Autodesk Inventor part; units mm, degrees
(part 6 of 8)
  spline S105 degree 3 poles (-3.7054, -6.6544) (-3.6945, -6.6546) (-3.6729, -6.6551) (-3.6415, -6.6595) (-3.6115, -6.6662) (-3.5832, -6.6758) (-3.5566, -6.6886) (-3.5316, -6.7039) (-3.5079, -6.7217) (-3.4866, -6.7426) (-3.467, -6.765) (-3.4501, -6.7888) (-3.4357, -6.8135) (-3.4236, -6.8391) (-3.4148, -6.8659) (-3.408, -6.8935) (-3.4042, -6.9223) (-3.4036, -6.9417) (-3.4033, -6.9516) knots 0 0 0 0 0.069475 0.136517 0.200789 0.26383 0.325735 0.387291 0.449509 0.512968 0.576275 0.63758 0.697903 0.757172 0.816599 0.876653 0.93729 1 1 1 1
  spline S106 degree 3 poles (-3.4033, -6.9516) (-3.4038, -6.9656) (-3.4048, -6.9932) (-3.413, -7.0337) (-3.4258, -7.0731) (-3.4412, -7.1047) (-3.4568, -7.1302) (-3.4708, -7.1512) (-3.4872, -7.1738) (-3.5063, -7.1979) (-3.5276, -7.2238) (-3.5513, -7.2514) (-3.5776, -7.2803) (-3.5961, -7.3001) (-3.6057, -7.3104) knots 0 0 0 0 0.098702 0.195672 0.292422 0.391343 0.444462 0.504229 0.570352 0.642546 0.722288 0.807921 0.90047 1 1 1 1
  line L71 (-3.6057, -7.3104) -> (-3.8559, -7.5774)
  line L72 (-3.8559, -7.5774) -> (-3.3905, -7.5774)
  line L73 (-3.3905, -7.5774) -> (-3.3905, -7.68)
  line L74 (-3.3905, -7.68) -> (-4.07, -7.68)
  line L75 (-4.07, -7.68) -> (-3.6822, -7.2661)
  spline S107 degree 3 poles (-3.6822, -7.2661) (-3.6727, -7.2563) (-3.6546, -7.2373) (-3.6289, -7.2097) (-3.6059, -7.1841) (-3.5853, -7.1605) (-3.5677, -7.1386) (-3.552, -7.1191) (-3.5394, -7.1012) (-3.5258, -7.0804) (-3.5126, -7.055) (-3.5012, -7.024) (-3.4943, -6.9921) (-3.4935, -6.9705) (-3.4931, -6.9596) knots 0 0 0 0 0.110803 0.212829 0.306101 0.390647 0.466924 0.534481 0.593587 0.644557 0.7362 0.825024 0.911986 1 1 1 1
  line L76 (-3.0444, -10.22) -> (-3.0572, -10.22)
  line L77 (-3.0572, -10.22) -> (-3.4803, -9.22)
  line L78 (-3.4803, -9.22) -> (-3.3841, -9.22)
  line L79 (-3.3841, -9.22) -> (-3.0508, -10.0081)
  line L80 (-3.0508, -10.0081) -> (-2.7174, -9.22)
  line L81 (-2.7174, -9.22) -> (-2.6213, -9.22)
  line L82 (-2.6213, -9.22) -> (-3.0444, -10.22)
  spline S108 degree 3 poles (-6.6469, -12.2726) (-6.6471, -12.285) (-6.6475, -12.3093) (-6.6506, -12.3452) (-6.6553, -12.3801) (-6.6624, -12.4137) (-6.6711, -12.4463) (-6.6822, -12.4777) (-6.695, -12.5081) (-6.7099, -12.5371) (-6.7262, -12.5645) (-6.7437, -12.5904) (-6.7624, -12.6143) (-6.7825, -12.6364) (-6.8036, -12.6566) (-6.826, -12.675) (-6.8496, -12.6913) (-6.8745, -12.7062) (-6.9013, -12.7192) (-6.9304, -12.7302) (-6.9622, -12.7393) (-6.9964, -12.7469) (-7.0331, -12.7529) (-7.0723, -12.7569) (-7.1141, -12.7596) (-7.1428, -12.7599) (-7.1575, -12.76) knots 0 0 0 0 0.046081 0.090807 0.134295 0.177024 0.218823 0.260244 0.30108 0.341614 0.381583 0.42012 0.458075 0.494738 0.531195 0.566934 0.602713 0.638327 0.674853 0.713467 0.754442 0.797815 0.843989 0.893072 0.944963 1 1 1 1
  line L83 (-7.1575, -12.76) -> (-7.4674, -12.76)
  line L84 (-7.4674, -12.76) -> (-7.4674, -11.76)
  line L85 (-7.4674, -11.76) -> (-7.2655, -11.76)
  spline S109 degree 3 poles (-7.2655, -11.76) (-7.248, -11.7601) (-7.214, -11.7604) (-7.165, -11.7619) (-7.1196, -11.7647) (-7.0781, -11.7687) (-7.0402, -11.7736) (-7.0062, -11.7797) (-6.9758, -11.7869) (-6.9571, -11.7931) (-6.9482, -11.7961) knots 0 0 0 0 0.164289 0.317406 0.458844 0.589367 0.707831 0.81577 0.91288 1 1 1 1
  spline S110 degree 3 poles (-6.9482, -11.7961) (-6.9366, -11.8005) (-6.9138, -11.8092) (-6.8812, -11.8256) (-6.8505, -11.8443) (-6.8216, -11.8651) (-6.7951, -11.8888) (-6.7699, -11.9142) (-6.7472, -11.9424) (-6.7264, -11.9727) (-6.7076, -12.0048) (-6.6913, -12.0386) (-6.6777, -12.0739) (-6.6664, -12.1107) (-6.6576, -12.1491) (-6.6515, -12.189) (-6.6475, -12.2303) (-6.6471, -12.2584) (-6.6469, -12.2726) knots 0 0 0 0 0.061545 0.121694 0.181155 0.239875 0.298702 0.357647 0.417605 0.478494 0.540407 0.602345 0.665004 0.728559 0.793651 0.860534 0.929236 1 1 1 1
  line L86 (-8.4033, -11.9747) -> (-8.4033, -12.76)
  line L87 (-8.4033, -12.76) -> (-8.4931, -12.76)
  line L88 (-8.4931, -12.76) -> (-8.4931, -11.76)
  line L89 (-8.4931, -11.76) -> (-8.4742, -11.76)
  line L90 (-8.4742, -11.76) -> (-7.8136, -12.5471)
  line L91 (-7.8136, -12.5471) -> (-7.8136, -11.76)
  line L92 (-7.8136, -11.76) -> (-7.7238, -11.76)
  line L93 (-7.7238, -11.76) -> (-7.7238, -12.76)
  line L94 (-7.7238, -12.76) -> (-7.7443, -12.76)
  line L95 (-7.7443, -12.76) -> (-8.4033, -11.9747)
  spline S111 degree 3 poles (-9.7495, -12.2596) (-9.7493, -12.2478) (-9.749, -12.2245) (-9.7454, -12.1898) (-9.7401, -12.1557) (-9.7324, -12.1222) (-9.7226, -12.0894) (-9.7105, -12.0572) (-9.6963, -12.0256) (-9.6799, -11.9948) (-9.6616, -11.9651) (-9.6417, -11.9369) (-9.62, -11.9104) (-9.5968, -11.8855) (-9.5718, -11.8624) (-9.5453, -11.841) (-9.5172, -11.8211) (-9.4875, -11.8031) (-9.4567, -11.7869) (-9.4246, -11.7728) (-9.3915, -11.7611) (-9.3575, -11.7511) (-9.3224, -11.7438) (-9.2864, -11.7384) (-9.2494, -11.7348) (-9.2243, -11.7345) (-9.2116, -11.7344) knots 0 0 0 0 0.042039 0.083544 0.124643 0.165303 0.206171 0.246971 0.288329 0.329987 0.371797 0.412738 0.453459 0.494001 0.534381 0.574952 0.615892 0.65725 0.699007 0.740486 0.782325 0.824567 0.867041 0.9105 0.954619 1 1 1 1
  spline S112 degree 3 poles (-9.2116, -11.7344) (-9.2013, -11.7345) (-9.1807, -11.7349) (-9.1502, -11.7371) (-9.1201, -11.7407) (-9.0905, -11.7457) (-9.0613, -11.7524) (-9.0327, -11.7604) (-9.0044, -11.7697) (-8.9766, -11.7809) (-8.9491, -11.7935) (-8.9218, -11.8077) (-8.8947, -11.8238) (-8.8679, -11.8417) (-8.841, -11.8613) (-8.8146, -11.8829) (-8.7881, -11.9058) (-8.771, -11.9223) (-8.7623, -11.9307) knots 0 0 0 0 0.061617 0.122179 0.182216 0.241864 0.30096 0.359969 0.419033 0.478069 0.537993 0.59896 0.661321 0.725248 0.79122 0.858746 0.928318 1 1 1 1
  line L96 (-8.7623, -11.9307) -> (-8.8392, -12.0036)
  spline S113 degree 3 poles (-8.8392, -12.0036) (-8.8532, -11.9905) (-8.8807, -11.9646) (-8.9255, -11.931) (-8.9723, -11.9023) (-9.0208, -11.8789) (-9.0698, -11.8602) (-9.1186, -11.8469) (-9.1668, -11.8384) (-9.1988, -11.8374) (-9.2146, -11.8369) knots 0 0 0 0 0.136144 0.269043 0.398517 0.5271 0.652283 0.77168 0.887495 1 1 1 1
  spline S114 degree 3 poles (-9.2146, -11.8369) (-9.2243, -11.837) (-9.2437, -11.8373) (-9.2724, -11.8403) (-9.3009, -11.8446) (-9.329, -11.8509) (-9.3568, -11.8588) (-9.3842, -11.8688) (-9.4112, -11.8804) (-9.4376, -11.8938) (-9.4633, -11.9085) (-9.4875, -11.9248) (-9.5105, -11.9421) (-9.5317, -11.961) (-9.5514, -11.9812) (-9.5699, -12.0024) (-9.5867, -12.0251) (-9.6019, -12.0489) (-9.6154, -12.0734) (-9.6274, -12.0984) (-9.6374, -12.1237) (-9.6453, -12.1495) (-9.6519, -12.1755) (-9.6565, -12.2018) (-9.6591, -12.2286) (-9.6595, -12.2466) (-9.6597, -12.2556) knots 0 0 0 0 0.042841 0.085571 0.127719 0.170068 0.212787 0.255482 0.298877 0.342861 0.386528 0.429532 0.471886 0.513729 0.555082 0.596535 0.63812 0.679822 0.721331 0.761888 0.802199 0.841806 0.88106 0.920633 0.960101 1 1 1 1
  spline S115 degree 3 poles (-9.6597, -12.2556) (-9.6595, -12.2648) (-9.6591, -12.2832) (-9.6563, -12.3107) (-9.6512, -12.3378) (-9.6444, -12.3645) (-9.6358, -12.391) (-9.6251, -12.4171) (-9.6125, -12.4428) (-9.5978, -12.4679) (-9.5818, -12.4923) (-9.5638, -12.5154) (-9.5447, -12.5373) (-9.5238, -12.5576) (-9.5017, -12.5768) (-9.4778, -12.5945) (-9.4526, -12.6109) (-9.4261, -12.6259) (-9.3984, -12.6393) (-9.3701, -12.6512) (-9.3409, -12.661) (-9.3111, -12.6689) (-9.2807, -12.6755) (-9.2496, -12.6797) (-9.2179, -12.6827) (-9.1965, -12.683) (-9.1858, -12.6831) knots 0 0 0 0 0.038994 0.077882 0.116652 0.155416 0.194618 0.234261 0.274547 0.315667 0.35702 0.398083 0.439098 0.479833 0.521274 0.562841 0.605292 0.648409 0.691727 0.735149 0.778369 0.821661 0.865524 0.909731 0.954523 1 1 1 1
  spline S116 degree 3 poles (-9.1858, -12.6831) (-9.1728, -12.6828) (-9.1474, -12.6823) (-9.1099, -12.6781) (-9.074, -12.6717) (-9.0396, -12.6622) (-9.0068, -12.6501) (-8.9754, -12.6355) (-8.9457, -12.6179) (-8.9175, -12.598) (-8.8916, -12.5759) (-8.8682, -12.552) (-8.8477, -12.5265) (-8.8299, -12.4994) (-8.8151, -12.4707) (-8.803, -12.4404) (-8.7937, -12.4085) (-8.7899, -12.3865) (-8.7879, -12.3754) knots 0 0 0 0 0.07063 0.138694 0.204918 0.269441 0.332636 0.395302 0.457764 0.520657 0.582852 0.643315 0.70258 0.760908 0.81949 0.878269 0.938491 1 1 1 1
  line L97 (-8.7879, -12.3754) -> (-9.1213, -12.3754)
  line L98 (-9.1213, -12.3754) -> (-9.1213, -12.2728)
  line L99 (-9.1213, -12.2728) -> (-8.6982, -12.2728)
  spline S117 degree 3 poles (-8.6982, -12.2728) (-8.6987, -12.2919) (-8.6996, -12.3294) (-8.7063, -12.3839) (-8.7171, -12.4354) (-8.7319, -12.484) (-8.751, -12.5295) (-8.7743, -12.572) (-8.802, -12.6113) (-8.8333, -12.6476) (-8.8684, -12.68) (-8.9064, -12.7084) (-8.9473, -12.7324) (-8.9912, -12.7519) (-9.0378, -12.7671) (-9.0872, -12.7779) (-9.1395, -12.7844) (-9.1753, -12.7852) (-9.1936, -12.7856) knots 0 0 0 0 0.071272 0.139493 0.204635 0.267406 0.328446 0.388397 0.447734 0.507392 0.566768 0.625478 0.684067 0.743248 0.804033 0.866499 0.931723 1 1 1 1
  spline S118 degree 3 poles (-9.1936, -12.7856) (-9.2049, -12.7855) (-9.2272, -12.7852) (-9.26, -12.7829) (-9.292, -12.7794) (-9.3231, -12.7741) (-9.3533, -12.7676) (-9.3827, -12.7593) (-9.4111, -12.7497) (-9.4388, -12.7387) (-9.4655, -12.726) (-9.4912, -12.7119) (-9.5161, -12.6965) (-9.5401, -12.6795) (-9.5633, -12.661) (-9.5855, -12.641) (-9.6068, -12.6195) (-9.6202, -12.6042) (-9.6269, -12.5965) knots 0 0 0 0 0.069237 0.136557 0.202094 0.266464 0.329769 0.391879 0.453271 0.514115 0.57439 0.634142 0.693923 0.754152 0.81447 0.875661 0.937348 1 1 1 1
  spline S119 degree 3 poles (-9.6269, -12.5965) (-9.6367, -12.5843) (-9.656, -12.5602) (-9.681, -12.5214) (-9.7022, -12.4813) (-9.7195, -12.4397) (-9.7329, -12.3967) (-9.7426, -12.3522) (-9.7483, -12.3064) (-9.7491, -12.2753) (-9.7495, -12.2596) knots 0 0 0 0 0.127896 0.253668 0.376738 0.499344 0.621999 0.745699 0.871345 1 1 1 1
  line L100 (-2.9033, -12.76) -> (-2.9033, -11.8626)
  line L101 (-2.9033, -11.8626) -> (-3.1213, -11.8626)
  line L102 (-3.1213, -11.8626) -> (-3.1213, -11.76)
  line L103 (-3.1213, -11.76) -> (-2.5956, -11.76)
  line L104 (-2.5956, -11.76) -> (-2.5956, -11.8626)
  line L105 (-2.5956, -11.8626) -> (-2.8136, -11.8626)
  line L106 (-2.8136, -11.8626) -> (-2.8136, -12.76)
  line L107 (-2.8136, -12.76) -> (-2.9033, -12.76)
  spline S120 degree 3 poles (-3.211, -12.515) (-3.2112, -12.524) (-3.2116, -12.5417) (-3.2159, -12.5678) (-3.2221, -12.5931) (-3.2316, -12.6174) (-3.2431, -12.641) (-3.2577, -12.6634) (-3.2746, -12.6851) (-3.2941, -12.7054) (-3.3154, -12.7241) (-3.3378, -12.7407) (-3.3616, -12.7546) (-3.3864, -12.7659) (-3.4124, -12.7747) (-3.4395, -12.7811) (-3.4677, -12.785) (-3.4869, -12.7854) (-3.4967, -12.7856) knots 0 0 0 0 0.061484 0.121775 0.18092 0.240256 0.300114 0.361146 0.423501 0.488669 0.553954 0.617581 0.680238 0.742187 0.804663 0.868259 0.93302 1 1 1 1
  spline S121 degree 3 poles (-3.4967, -12.7856) (-3.5042, -12.7855) (-3.5192, -12.7852) (-3.5414, -12.7826) (-3.5632, -12.779) (-3.5842, -12.7732) (-3.6048, -12.7663) (-3.6249, -12.7576) (-3.6444, -12.7473) (-3.6635, -12.7355) (-3.6821, -12.7218) (-3.7001, -12.7058) (-3.718, -12.688) (-3.7353, -12.6679) (-3.7524, -12.6458) (-3.769, -12.6215) (-3.7853, -12.5952) (-3.7955, -12.5766) (-3.8008, -12.5671) knots 0 0 0 0 0.057208 0.113696 0.169178 0.224159 0.27872 0.333794 0.389241 0.445822 0.503704 0.564294 0.627975 0.695038 0.765373 0.839611 0.917538 1 1 1 1
  line L108 (-3.8008, -12.5671) -> (-3.7162, -12.5164)
  spline S122 degree 3 poles (-3.7162, -12.5164) (-3.7084, -12.5296) (-3.6933, -12.5548) (-3.6682, -12.5889) (-3.6421, -12.6178) (-3.615, -12.6415) (-3.5869, -12.6601) (-3.5577, -12.6733) (-3.5275, -12.6816) (-3.5069, -12.6826) (-3.4967, -12.6831) knots 0 0 0 0 0.159004 0.304646 0.438547 0.562322 0.677433 0.786897 0.893611 1 1 1 1
  spline S123 degree 3 poles (-3.4967, -12.6831) (-3.4879, -12.6828) (-3.4705, -12.6823) (-3.4449, -12.6777) (-3.4201, -12.6706) (-3.3965, -12.6603) (-3.3745, -12.6479) (-3.3551, -12.633) (-3.3384, -12.6162) (-3.3248, -12.5976) (-3.3143, -12.5775) (-3.3063, -12.5568) (-3.3018, -12.5354) (-3.3011, -12.5209) (-3.3008, -12.5136) knots 0 0 0 0 0.091264 0.18093 0.270088 0.360156 0.448343 0.532666 0.613834 0.693982 0.772716 0.849335 0.923967 1 1 1 1
  spline S124 degree 3 poles (-3.3008, -12.5136) (-3.3012, -12.5053) (-3.302, -12.4884) (-3.3093, -12.4634) (-3.3207, -12.4387) (-3.3312, -12.4234) (-3.3366, -12.4154) knots 0 0 0 0 0.234723 0.477158 0.728556 1 1 1 1
  spline S125 degree 3 poles (-3.3366, -12.4154) (-3.3411, -12.4097) (-3.3505, -12.3977) (-3.3667, -12.3798) (-3.3856, -12.3613) (-3.4067, -12.3416) (-3.4308, -12.3215) (-3.457, -12.3001) (-3.486, -12.2782) (-3.5064, -12.2636) (-3.5169, -12.256) knots 0 0 0 0 0.090279 0.18953 0.299198 0.418926 0.548376 0.688136 0.839084 1 1 1 1
  spline S126 degree 3 poles (-3.5169, -12.256) (-3.5274, -12.2485) (-3.5476, -12.2342) (-3.5757, -12.2129) (-3.6008, -12.1935) (-3.6229, -12.1757) (-3.6419, -12.1595) (-3.6579, -12.1451) (-3.6706, -12.1322) (-3.6776, -12.1238) (-3.6808, -12.12) knots 0 0 0 0 0.181535 0.347082 0.495568 0.628357 0.74552 0.845831 0.930782 1 1 1 1
  spline S127 degree 3 poles (-3.6808, -12.12) (-3.6852, -12.1141) (-3.6939, -12.1025) (-3.7054, -12.0844) (-3.7151, -12.0659) (-3.7228, -12.0469) (-3.7292, -12.0277) (-3.7335, -12.008) (-3.7362, -11.988) (-3.7365, -11.9745) (-3.7367, -11.9677) knots 0 0 0 0 0.133507 0.262559 0.388264 0.512667 0.633722 0.755394 0.877553 1 1 1 1
  spline S128 degree 3 poles (-3.7367, -11.9677) (-3.7363, -11.9572) (-3.7356, -11.9362) (-3.7293, -11.9056) (-3.7195, -11.8764) (-3.7057, -11.8489) (-3.6879, -11.8238) (-3.6673, -11.8008) (-3.6428, -11.7814) (-3.6159, -11.7645) (-3.5864, -11.7512) (-3.5556, -11.7412) (-3.5233, -11.7356) (-3.5014, -11.7348) (-3.4903, -11.7344) knots 0 0 0 0 0.083785 0.16578 0.24628 0.327461 0.408797 0.489715 0.571376 0.655523 0.741019 0.826547 0.911989 1 1 1 1
  spline S129 degree 3 poles (-3.4903, -11.7344) (-3.4785, -11.7348) (-3.4551, -11.7356) (-3.4206, -11.7426) (-3.3874, -11.7542) (-3.3607, -11.7674) (-3.3398, -11.7806) (-3.3239, -11.7926) (-3.3077, -11.8064) (-3.2912, -11.8221) (-3.2747, -11.8398) (-3.2578, -11.8593) (-3.2406, -11.8806) (-3.2295, -11.8958) (-3.2238, -11.9036) knots 0 0 0 0 0.107233 0.213252 0.31883 0.426794 0.483646 0.543604 0.608308 0.677127 0.750686 0.828713 0.91219 1 1 1 1
  line L109 (-3.2238, -11.9036) -> (-3.305, -11.9651)
  spline S130 degree 3 poles (-3.305, -11.9651) (-3.3099, -11.9588) (-3.3193, -11.9467) (-3.3336, -11.9296) (-3.3471, -11.9141) (-3.3604, -11.9006) (-3.3728, -11.8884) (-3.3849, -11.8779) (-3.3964, -11.8692) (-3.4108, -11.8598) (-3.4291, -11.8505) (-3.4519, -11.8426) (-3.4758, -11.8379) (-3.4921, -11.8372) (-3.5003, -11.8369) knots 0 0 0 0 0.098469 0.189629 0.274184 0.352183 0.423199 0.488551 0.548473 0.60144 0.701198 0.799592 0.898545 1 1 1 1
  spline S131 degree 3 poles (-3.5003, -11.8369) (-3.5106, -11.8373) (-3.5305, -11.8379) (-3.5588, -11.8452) (-3.5843, -11.8567) (-3.6062, -11.8728) (-3.6244, -11.8919) (-3.6375, -11.9138) (-3.6455, -11.938) (-3.6464, -11.9549) (-3.6469, -11.9635) knots 0 0 0 0 0.143073 0.275903 0.402371 0.528414 0.650356 0.765895 0.880774 1 1 1 1
  spline S132 degree 3 poles (-3.6469, -11.9635) (-3.6468, -11.9689) (-3.6466, -11.9796) (-3.6435, -11.9955) (-3.6394, -12.0113) (-3.633, -12.0269) (-3.6242, -12.0428) (-3.6127, -12.0591) (-3.5981, -12.076) (-3.5869, -12.0869) (-3.581, -12.0927) knots 0 0 0 0 0.107285 0.214746 0.322939 0.434116 0.553412 0.686073 0.834256 1 1 1 1
  spline S133 degree 3 poles (-3.581, -12.0927) (-3.5788, -12.0947) (-3.5736, -12.0993) (-3.5641, -12.1069) (-3.5516, -12.1163) (-3.5363, -12.1279) (-3.518, -12.1413) (-3.4967, -12.1565) (-3.4727, -12.1738) (-3.4556, -12.1859) (-3.4466, -12.1923) knots 0 0 0 0 0.052594 0.124952 0.218094 0.333502 0.468789 0.624938 0.801683 1 1 1 1
  spline S134 degree 3 poles (-3.4466, -12.1923) (-3.4357, -12.2002) (-3.4147, -12.2155) (-3.3848, -12.2385) (-3.3577, -12.2609) (-3.3333, -12.2828) (-3.3113, -12.3038) (-3.2921, -12.3242) (-3.2753, -12.3439) (-3.2572, -12.3693) (-3.2388, -12.4003) (-3.223, -12.4384) (-3.213, -12.4766) (-3.2117, -12.5023) (-3.211, -12.515) knots 0 0 0 0 0.096972 0.187773 0.272396 0.351321 0.424335 0.491909 0.554233 0.611268 0.716348 0.81454 0.908495 1 1 1 1
  spline S135 degree 3 poles (4.429, 5.5196) (4.4288, 5.5043) (4.4284, 5.4745) (4.4265, 5.4309) (4.4228, 5.3898) (4.4182, 5.351) (4.4118, 5.3147) (4.4039, 5.2808) (4.3952, 5.2491) (4.3843, 5.2198) (4.3725, 5.1927) (4.3596, 5.1674) (4.3458, 5.1436) (4.3308, 5.1216) (4.3148, 5.1012) (4.2975, 5.0828) (4.2793, 5.0659) (4.26, 5.0509) (4.2399, 5.0377) (4.2193, 5.0259) (4.198, 5.0164) (4.1763, 5.0083) (4.154, 5.002) (4.131, 4.9977) (4.1076, 4.9947) (4.0918, 4.9945) (4.0838, 4.9944) knots 0 0 0 0 0.065063 0.126773 0.185516 0.240765 0.29298 0.34225 0.388919 0.432776 0.474628 0.514775 0.553606 0.591426 0.628028 0.663804 0.698984 0.733591 0.767628 0.801208 0.834264 0.866981 0.89972 0.932702 0.966176 1 1 1 1
  spline S136 degree 3 poles (4.0838, 4.9944) (4.0759, 4.9945) (4.0604, 4.9948) (4.0373, 4.9975) (4.015, 5.0018) (3.9932, 5.008) (3.9718, 5.0155) (3.9512, 5.0252) (3.9311, 5.0364) (3.9116, 5.0492) (3.8931, 5.0639) (3.8753, 5.0801) (3.8589, 5.0983) (3.8435, 5.1182) (3.829, 5.1395) (3.8156, 5.1626) (3.8032, 5.1874) (3.7919, 5.2141) (3.7818, 5.243) (3.7729, 5.2745) (3.7659, 5.3088) (3.7599, 5.3457) (3.7551, 5.3853) (3.7518, 5.4277) (3.7498, 5.4728) (3.7496, 5.5037) (3.7495, 5.5196) knots 0 0 0 0 0.033787 0.066622 0.099285 0.131361 0.163585 0.196104 0.228902 0.262158 0.295991 0.330218 0.36506 0.400951 0.43762 0.475708 0.515381 0.556414 0.599765 0.646424 0.696431 0.749782 0.806573 0.867436 0.931887 1 1 1 1
  spline S137 degree 3 poles (3.7495, 5.5196) (3.7496, 5.5356) (3.7498, 5.5668) (3.7518, 5.6121) (3.7552, 5.6547) (3.7598, 5.6944) (3.7654, 5.7314) (3.7729, 5.7655) (3.7814, 5.7968) (3.7913, 5.8255) (3.8024, 5.852) (3.8145, 5.8766) (3.8281, 5.8995) (3.8424, 5.921) (3.8579, 5.9407) (3.8743, 5.9589) (3.8921, 5.9751) (3.9108, 5.99) (3.9306, 6.0029) (3.9507, 6.0144) (3.9715, 6.0241) (3.993, 6.0318) (4.0149, 6.0382) (4.0373, 6.0425) (4.0604, 6.0452) (4.0759, 6.0455) (4.0838, 6.0456) knots 0 0 0 0 0.068595 0.133246 0.194313 0.251279 0.304513 0.354235 0.400481 0.443411 0.484015 0.523252 0.561042 0.5979 0.633518 0.668314 0.702496 0.736685 0.770293 0.803437 0.835913 0.86846 0.900847 0.933467 0.966258 1 1 1 1
  spline S138 degree 3 poles (4.0838, 6.0456) (4.0918, 6.0455) (4.1076, 6.0452) (4.131, 6.0426) (4.1538, 6.0381) (4.176, 6.0319) (4.1978, 6.0241) (4.2189, 6.0144) (4.2395, 6.003) (4.2593, 5.9897) (4.2785, 5.9749) (4.2967, 5.9581) (4.3137, 5.9395) (4.3299, 5.9194) (4.3448, 5.8973) (4.359, 5.8737) (4.3716, 5.848) (4.3838, 5.8208) (4.3944, 5.7913) (4.4039, 5.7597) (4.4116, 5.7255) (4.418, 5.689) (4.4229, 5.65) (4.4265, 5.6087) (4.4284, 5.5649) (4.4288, 5.535) (4.429, 5.5196) knots 0 0 0 0 0.033788 0.067194 0.099862 0.132567 0.165151 0.197913 0.231319 0.265083 0.299255 0.334399 0.369943 0.406284 0.444064 0.482998 0.523354 0.565537 0.609613 0.656391 0.705885 0.758325 0.813832 0.872795 0.934722 1 1 1 1
  line L110 (4.9674, 5.02) -> (4.9546, 5.02)
  line L111 (4.9546, 5.02) -> (4.5315, 6.02)
  line L112 (4.5315, 6.02) -> (4.6277, 6.02)
  line L113 (4.6277, 6.02) -> (4.961, 5.2319)
  line L114 (4.961, 5.2319) -> (5.2944, 6.02)
  line L115 (5.2944, 6.02) -> (5.3905, 6.02)
  line L116 (5.3905, 6.02) -> (4.9674, 5.02)
  spline S139 degree 3 poles (5.7495, 2.9674) (5.7493, 2.955) (5.749, 2.9307) (5.7458, 2.8948) (5.7412, 2.8599) (5.734, 2.8263) (5.7253, 2.7937) (5.7142, 2.7623) (5.7014, 2.7319) (5.6866, 2.7029) (5.6702, 2.6755) (5.6527, 2.6496) (5.634, 2.6257) (5.614, 2.6036) (5.5928, 2.5834) (5.5704, 2.565) (5.5468, 2.5487) (5.5219, 2.5338) (5.4951, 2.5208) (5.466, 2.5098) (5.4342, 2.5007) (5.4001, 2.4931) (5.3633, 2.4871) (5.3241, 2.4831) (5.2823, 2.4804) (5.2536, 2.4801) (5.2389, 2.48) knots 0 0 0 0 0.046081 0.090807 0.134295 0.177024 0.218823 0.260244 0.30108 0.341614 0.381583 0.42012 0.458075 0.494738 0.531195 0.566934 0.602713 0.638327 0.674853 0.713467 0.754442 0.797815 0.843989 0.893072 0.944963 1 1 1 1
  line L117 (5.2389, 2.48) -> (4.929, 2.48)
  line L118 (4.929, 2.48) -> (4.929, 3.48)
  line L119 (4.929, 3.48) -> (5.1309, 3.48)
  spline S140 degree 3 poles (5.1309, 3.48) (5.1485, 3.4799) (5.1824, 3.4796) (5.2314, 3.4781) (5.2768, 3.4753) (5.3183, 3.4713) (5.3562, 3.4664) (5.3902, 3.4603) (5.4207, 3.4531) (5.4394, 3.4469) (5.4482, 3.4439) knots 0 0 0 0 0.164289 0.317406 0.458844 0.589367 0.707831 0.81577 0.91288 1 1 1 1
  spline S141 degree 3 poles (5.4482, 3.4439) (5.4598, 3.4395) (5.4827, 3.4308) (5.5152, 3.4144) (5.5459, 3.3957) (5.5748, 3.3749) (5.6013, 3.3512) (5.6265, 3.3258) (5.6492, 3.2976) (5.67, 3.2673) (5.6888, 3.2352) (5.7052, 3.2014) (5.7187, 3.1661) (5.73, 3.1293) (5.7388, 3.0909) (5.7449, 3.051) (5.7489, 3.0097) (5.7493, 2.9816) (5.7495, 2.9674) knots 0 0 0 0 0.061545 0.121694 0.181155 0.239875 0.298702 0.357647 0.417605 0.478494 0.540407 0.602345 0.665004 0.728559 0.793651 0.860534 0.929236 1 1 1 1
  spline S142 degree 3 poles (8.0572, 2.9796) (8.057, 2.9643) (8.0566, 2.9345) (8.0548, 2.8909) (8.051, 2.8498) (8.0464, 2.811) (8.04, 2.7747) (8.0321, 2.7408) (8.0234, 2.7091) (8.0125, 2.6798) (8.0007, 2.6527) (7.9878, 2.6274) (7.9741, 2.6036) (7.959, 2.5816) (7.943, 2.5612) (7.9257, 2.5428) (7.9075, 2.5259) (7.8882, 2.5109) (7.8681, 2.4977) (7.8475, 2.4859) (7.8262, 2.4764) (7.8045, 2.4683) (7.7822, 2.462) (7.7592, 2.4577) (7.7358, 2.4547) (7.72, 2.4545) (7.712, 2.4544) knots 0 0 0 0 0.065063 0.126773 0.185516 0.240765 0.29298 0.34225 0.388919 0.432776 0.474628 0.514775 0.553606 0.591426 0.628028 0.663804 0.698984 0.733591 0.767628 0.801208 0.834264 0.866981 0.89972 0.932702 0.966176 1 1 1 1
  spline S143 degree 3 poles (7.712, 2.4544) (7.7041, 2.4545) (7.6886, 2.4548) (7.6655, 2.4575) (7.6432, 2.4618) (7.6214, 2.468) (7.6, 2.4755) (7.5794, 2.4852) (7.5594, 2.4964) (7.5398, 2.5092) (7.5213, 2.5239) (7.5035, 2.5401) (7.4871, 2.5583) (7.4717, 2.5782) (7.4572, 2.5995) (7.4438, 2.6226) (7.4314, 2.6474) (7.4201, 2.6741) (7.41, 2.703) (7.4011, 2.7345) (7.3941, 2.7688) (7.3881, 2.8057) (7.3833, 2.8453) (7.38, 2.8877) (7.378, 2.9328) (7.3778, 2.9637) (7.3777, 2.9796) knots 0 0 0 0 0.033787 0.066622 0.099285 0.131361 0.163585 0.196104 0.228902 0.262158 0.295991 0.330218 0.36506 0.400951 0.43762 0.475708 0.515381 0.556414 0.599765 0.646424 0.696431 0.749782 0.806573 0.867436 0.931887 1 1 1 1
  spline S144 degree 3 poles (7.3777, 2.9796) (7.3778, 2.9956) (7.378, 3.0268) (7.38, 3.0721) (7.3834, 3.1147) (7.388, 3.1544) (7.3936, 3.1914) (7.4011, 3.2255) (7.4096, 3.2568) (7.4195, 3.2855) (7.4306, 3.312) (7.4427, 3.3366) (7.4563, 3.3595) (7.4706, 3.381) (7.4861, 3.4007) (7.5025, 3.4189) (7.5203, 3.4351) (7.539, 3.45) (7.5588, 3.4629) (7.5789, 3.4744) (7.5997, 3.4841) (7.6212, 3.4918) (7.6431, 3.4982) (7.6655, 3.5025) (7.6886, 3.5052) (7.7041, 3.5055) (7.712, 3.5056) knots 0 0 0 0 0.068595 0.133246 0.194313 0.251279 0.304513 0.354235 0.400481 0.443411 0.484015 0.523252 0.561042 0.5979 0.633518 0.668314 0.702496 0.736685 0.770293 0.803437 0.835913 0.86846 0.900847 0.933467 0.966258 1 1 1 1
  spline S145 degree 3 poles (7.712, 3.5056) (7.72, 3.5055) (7.7358, 3.5052) (7.7592, 3.5026) (7.782, 3.4981) (7.8042, 3.4919) (7.826, 3.4841) (7.8471, 3.4744) (7.8677, 3.463) (7.8875, 3.4497) (7.9067, 3.4349) (7.9249, 3.4181) (7.9419, 3.3995) (7.9581, 3.3794) (7.973, 3.3573) (7.9872, 3.3337) (7.9998, 3.308) (8.012, 3.2808) (8.0226, 3.2513) (8.0321, 3.2197) (8.0398, 3.1855) (8.0462, 3.149) (8.0511, 3.11) (8.0547, 3.0687) (8.0566, 3.0249) (8.057, 2.995) (8.0572, 2.9796) knots 0 0 0 0 0.033788 0.067194 0.099862 0.132567 0.165151 0.197913 0.231319 0.265083 0.299255 0.334399 0.369943 0.406284 0.444064 0.482998 0.523354 0.565537 0.609613 0.656391 0.705885 0.758325 0.813832 0.872795 0.934722 1 1 1 1
  line L120 (2.9162, 0.8374) -> (2.7623, 0.8374)
  line L121 (2.7623, 0.8374) -> (2.821, 0.94)
  line L122 (2.821, 0.94) -> (3.0059, 0.94)
  line L123 (3.0059, 0.94) -> (3.0059, -0.06)
  line L124 (3.0059, -0.06) -> (2.9162, -0.06)
  line L125 (2.9162, -0.06) -> (2.9162, 0.8374)
  spline S146 degree 3 poles (7.2879, 0.4396) (7.2878, 0.4243) (7.2874, 0.3945) (7.2855, 0.3509) (7.2818, 0.3098) (7.2772, 0.271) (7.2708, 0.2347) (7.2629, 0.2008) (7.2541, 0.1691) (7.2433, 0.1398) (7.2315, 0.1127) (7.2186, 0.0874) (7.2048, 0.0636) (7.1898, 0.0416) (7.1738, 0.0212) (7.1564, 0.0028) (7.1382, -0.0141) (7.119, -0.0291) (7.0989, -0.0423) (7.0783, -0.0541) (7.0569, -0.0636) (7.0352, -0.0717) (7.0129, -0.078) (6.99, -0.0823) (6.9666, -0.0853) (6.9508, -0.0855) (6.9428, -0.0856) knots 0 0 0 0 0.065063 0.126773 0.185516 0.240765 0.29298 0.34225 0.388919 0.432776 0.474628 0.514775 0.553606 0.591426 0.628028 0.663804 0.698984 0.733591 0.767628 0.801208 0.834264 0.866981 0.89972 0.932702 0.966176 1 1 1 1
  spline S147 degree 3 poles (6.9428, -0.0856) (6.9349, -0.0855) (6.9194, -0.0852) (6.8963, -0.0825) (6.8739, -0.0782) (6.8521, -0.072) (6.8308, -0.0645) (6.8102, -0.0548) (6.7901, -0.0436) (6.7706, -0.0308) (6.752, -0.0161) (6.7343, 0.0001) (6.7178, 0.0183) (6.7025, 0.0382) (6.6879, 0.0595) (6.6745, 0.0826) (6.6622, 0.1074) (6.6508, 0.1341) (6.6408, 0.163) (6.6319, 0.1945) (6.6249, 0.2288) (6.6189, 0.2657) (6.6141, 0.3053) (6.6108, 0.3477) (6.6087, 0.3928) (6.6086, 0.4237) (6.6085, 0.4396) knots 0 0 0 0 0.033787 0.066622 0.099285 0.131361 0.163585 0.196104 0.228902 0.262158 0.295991 0.330218 0.36506 0.400951 0.43762 0.475708 0.515381 0.556414 0.599765 0.646424 0.696431 0.749782 0.806573 0.867436 0.931887 1 1 1 1
  spline S148 degree 3 poles (6.6085, 0.4396) (6.6086, 0.4556) (6.6087, 0.4868) (6.6108, 0.5321) (6.6141, 0.5747) (6.6187, 0.6144) (6.6243, 0.6514) (6.6318, 0.6855) (6.6404, 0.7168) (6.6502, 0.7455) (6.6614, 0.772) (6.6735, 0.7966) (6.6871, 0.8195) (6.7014, 0.841) (6.7169, 0.8607) (6.7333, 0.8789) (6.7511, 0.8951) (6.7698, 0.91) (6.7895, 0.9229) (6.8097, 0.9344) (6.8305, 0.9441) (6.8519, 0.9518) (6.8739, 0.9582) (6.8963, 0.9625) (6.9194, 0.9652) (6.9349, 0.9655) (6.9428, 0.9656) knots 0 0 0 0 0.068595 0.133246 0.194313 0.251279 0.304513 0.354235 0.400481 0.443411 0.484015 0.523252 0.561042 0.5979 0.633518 0.668314 0.702496 0.736685 0.770293 0.803437 0.835913 0.86846 0.900847 0.933467 0.966258 1 1 1 1
  spline S149 degree 3 poles (6.9428, 0.9656) (6.9507, 0.9655) (6.9666, 0.9652) (6.9899, 0.9626) (7.0128, 0.9581) (7.035, 0.9519) (7.0567, 0.9441) (7.0779, 0.9344) (7.0985, 0.923) (7.1183, 0.9097) (7.1375, 0.8949) (7.1556, 0.8781) (7.1727, 0.8595) (7.1889, 0.8394) (7.2038, 0.8173) (7.2179, 0.7937) (7.2306, 0.768) (7.2428, 0.7408) (7.2534, 0.7113) (7.2629, 0.6797) (7.2705, 0.6455) (7.2769, 0.609) (7.2819, 0.57) (7.2855, 0.5287) (7.2874, 0.4849) (7.2878, 0.455) (7.2879, 0.4396) knots 0 0 0 0 0.033788 0.067194 0.099862 0.132567 0.165151 0.197913 0.231319 0.265083 0.299255 0.334399 0.369943 0.406284 0.444064 0.482998 0.523354 0.565537 0.609613 0.656391 0.705885 0.758325 0.813832 0.872795 0.934722 1 1 1 1
  line L126 (2.7879, -10.22) -> (2.6982, -10.22)
  line L127 (2.6982, -10.22) -> (2.6982, -9.22)
  line L128 (2.6982, -9.22) -> (2.8983, -9.22)
  spline S150 degree 3 poles (2.8983, -9.22) (2.9117, -9.22) (2.9373, -9.2201) (2.9741, -9.2206) (3.0074, -9.222) (3.0374, -9.2231) (3.0641, -9.2253) (3.0874, -9.2273) (3.1074, -9.23) (3.1194, -9.2325) (3.1249, -9.2336) knots 0 0 0 0 0.176258 0.338434 0.484822 0.617158 0.734698 0.837385 0.926372 1 1 1 1
  spline S151 degree 3 poles (3.1249, -9.2336) (3.1322, -9.2354) (3.1467, -9.239) (3.1675, -9.2466) (3.1874, -9.2553) (3.2062, -9.2656) (3.2238, -9.2775) (3.2405, -9.2907) (3.2562, -9.3053) (3.2705, -9.3216) (3.2839, -9.3387) (3.2952, -9.3572) (3.3049, -9.3766) (3.3127, -9.3969) (3.319, -9.4181) (3.3234, -9.4404) (3.326, -9.4636) (3.3263, -9.4794) (3.3264, -9.4874) knots 0 0 0 0 0.064217 0.127064 0.188745 0.249132 0.309453 0.369827 0.43065 0.492352 0.554072 0.61569 0.676798 0.738439 0.801317 0.865185 0.931641 1 1 1 1
  spline S152 degree 3 poles (3.3264, -9.4874) (3.326, -9.5008) (3.3252, -9.5268) (3.3175, -9.5645) (3.305, -9.5997) (3.2878, -9.6323) (3.2658, -9.6617) (3.2395, -9.6875) (3.2086, -9.7091) (3.1799, -9.7241) (3.1546, -9.7337) (3.1337, -9.7405) (3.111, -9.7457) (3.0865, -9.7504) (3.0603, -9.7539) (3.0324, -9.7565) (3.0027, -9.7581) (2.9823, -9.7583) (2.9718, -9.7585) knots 0 0 0 0 0.07878 0.153721 0.226714 0.299191 0.37119 0.443006 0.516689 0.593217 0.633873 0.676989 0.7229 0.771959 0.824211 0.879379 0.937948 1 1 1 1
  line L129 (2.9718, -9.7585) -> (3.3392, -10.22)
  line L130 (3.3392, -10.22) -> (3.2283, -10.22)
  line L131 (3.2283, -10.22) -> (2.8609, -9.7585)
  line L132 (2.8609, -9.7585) -> (2.7879, -9.7585)
  line L133 (2.7879, -9.7585) -> (2.7879, -10.22)
  line L134 (3.461, -10.22) -> (3.7875, -9.71)
  line L135 (3.7875, -9.71) -> (3.4738, -9.22)
  line L136 (3.4738, -9.22) -> (3.5774, -9.22)
  line L137 (3.5774, -9.22) -> (3.8392, -9.6291)
  line L138 (3.8392, -9.6291) -> (4.101, -9.22)
  line L139 (4.101, -9.22) -> (4.2046, -9.22)
  line L140 (4.2046, -9.22) -> (3.8911, -9.71)
  line L141 (3.8911, -9.71) -> (4.2174, -10.22)
  line L142 (4.2174, -10.22) -> (4.1139, -10.22)
  line L143 (4.1139, -10.22) -> (3.8392, -9.7909)
  line L144 (3.8392, -9.7909) -> (3.5646, -10.22)
  line L145 (3.5646, -10.22) -> (3.461, -10.22)
  spline S153 degree 3 poles (7.1854, -9.4996) (7.1852, -9.4928) (7.1848, -9.4794) (7.1817, -9.4597) (7.1769, -9.4406) (7.1701, -9.4223) (7.161, -9.4047) (7.15, -9.388) (7.1374, -9.3718) (7.1227, -9.3566) (7.1066, -9.3427) (7.0895, -9.3303) (7.0715, -9.32) (7.0526, -9.3116) (7.0328, -9.305) (7.0121, -9.3004) (6.9906, -9.2975) (6.9759, -9.2971) (6.9684, -9.2969) knots 0 0 0 0 0.061965 0.122122 0.180988 0.239933 0.299906 0.359989 0.421776 0.486576 0.551535 0.615018 0.677259 0.73973 0.80305 0.866495 0.931973 1 1 1 1
  spline S154 degree 3 poles (6.9684, -9.2969) (6.9606, -9.2971) (6.9453, -9.2975) (6.9227, -9.3003) (6.9012, -9.3052) (6.8807, -9.3118) (6.8611, -9.3202) (6.8426, -9.3307) (6.8251, -9.3432) (6.8087, -9.3574) (6.7936, -9.3732) (6.7804, -9.3908) (6.7688, -9.4099) (6.7586, -9.4304) (6.7504, -9.4526) (6.7441, -9.4763) (6.7392, -9.5014) (6.7375, -9.5188) (6.7367, -9.5277) knots 0 0 0 0 0.064439 0.126547 0.186887 0.245878 0.304041 0.362191 0.420976 0.48066 0.5406 0.600689 0.661936 0.724443 0.789038 0.856314 0.926352 1 1 1 1
  line L146 (6.7367, -9.5277) -> (6.6469, -9.5277)
  spline S155 degree 3 poles (6.6469, -9.5277) (6.6475, -9.5158) (6.6487, -9.4924) (6.654, -9.4583) (6.6617, -9.4257) (6.6726, -9.3949) (6.6861, -9.3656) (6.7023, -9.3379) (6.7215, -9.3119) (6.7433, -9.2878) (6.767, -9.2658) (6.7925, -9.2467) (6.8193, -9.2306) (6.8473, -9.2172) (6.8769, -9.2071) (6.9077, -9.1996) (6.9399, -9.1951) (6.9619, -9.1946) (6.973, -9.1944) knots 0 0 0 0 0.068791 0.135103 0.198979 0.261904 0.323495 0.385195 0.446969 0.509765 0.572251 0.633405 0.693251 0.752583 0.812579 0.873275 0.93555 1 1 1 1
  spline S156 degree 3 poles (6.973, -9.1944) (6.984, -9.1946) (7.0056, -9.1951) (7.037, -9.1995) (7.0669, -9.2062) (7.0953, -9.2158) (7.1219, -9.2286) (7.1469, -9.2439) (7.1705, -9.2617) (7.1919, -9.2826) (7.2114, -9.305) (7.2283, -9.3288) (7.2428, -9.3535) (7.2548, -9.3791) (7.2637, -9.4059) (7.2704, -9.4335) (7.2742, -9.4623) (7.2748, -9.4817) (7.2751, -9.4916) knots 0 0 0 0 0.069475 0.136517 0.200789 0.26383 0.325735 0.387291 0.449509 0.512968 0.576275 0.63758 0.697903 0.757172 0.816599 0.876653 0.93729 1 1 1 1
  spline S157 degree 3 poles (7.2751, -9.4916) (7.2746, -9.5056) (7.2737, -9.5332) (7.2655, -9.5737) (7.2527, -9.6131) (7.2372, -9.6447) (7.2217, -9.6702) (7.2077, -9.6912) (7.1912, -9.7138) (7.1722, -9.7379) (7.1509, -9.7638) (7.1272, -9.7914) (7.1009, -9.8203) (7.0824, -9.8401) (7.0728, -9.8504) knots 0 0 0 0 0.098702 0.195672 0.292422 0.391343 0.444462 0.504229 0.570352 0.642546 0.722288 0.807921 0.90047 1 1 1 1
  line L147 (7.0728, -9.8504) -> (6.8226, -10.1174)
  line L148 (6.8226, -10.1174) -> (7.2879, -10.1174)
  line L149 (7.2879, -10.1174) -> (7.2879, -10.22)
  line L150 (7.2879, -10.22) -> (6.6085, -10.22)
  line L151 (6.6085, -10.22) -> (6.9963, -9.8061)
  spline S158 degree 3 poles (6.9963, -9.8061) (7.0057, -9.7963) (7.0239, -9.7773) (7.0495, -9.7497) (7.0726, -9.7241) (7.0931, -9.7005) (7.1108, -9.6786) (7.1265, -9.6591) (7.139, -9.6412) (7.1527, -9.6204) (7.1659, -9.595) (7.1772, -9.564) (7.1841, -9.5321) (7.185, -9.5105) (7.1854, -9.4996) knots 0 0 0 0 0.110803 0.212829 0.306101 0.390647 0.466924 0.534481 0.593587 0.644557 0.7362 0.825024 0.911986 1 1 1 1
  line L152 (7.9053, -9.3226) -> (7.4418, -9.3226)
  line L153 (7.4418, -9.3226) -> (7.4418, -9.22)
  line L154 (7.4418, -9.22) -> (8.0572, -9.22)
  line L155 (8.0572, -9.22) -> (7.5315, -10.2456)
  line L156 (7.5315, -10.2456) -> (7.454, -10.203)
  line L157 (7.454, -10.203) -> (7.9053, -9.3226)
  spline S159 degree 3 poles (6.6469, -12.2596) (6.6471, -12.2478) (6.6474, -12.2245) (6.651, -12.1898) (6.6563, -12.1557) (6.664, -12.1222) (6.6738, -12.0894) (6.6859, -12.0572) (6.7001, -12.0256) (6.7165, -11.9948) (6.7348, -11.9651) (6.7547, -11.9369) (6.7764, -11.9104) (6.7996, -11.8855) (6.8246, -11.8624) (6.8511, -11.841) (6.8792, -11.8211) (6.9089, -11.8031) (6.9398, -11.7869) (6.9718, -11.7728) (7.0049, -11.7611) (7.0389, -11.7511) (7.074, -11.7438) (7.11, -11.7384) (7.147, -11.7348) (7.1721, -11.7345) (7.1848, -11.7344) knots 0 0 0 0 0.042039 0.083544 0.124643 0.165303 0.206171 0.246971 0.288329 0.329987 0.371797 0.412738 0.453459 0.494001 0.534381 0.574952 0.615892 0.65725 0.699007 0.740486 0.782325 0.824567 0.867041 0.9105 0.954619 1 1 1 1
  spline S160 degree 3 poles (7.1848, -11.7344) (7.1951, -11.7345) (7.2157, -11.7349) (7.2462, -11.7371) (7.2763, -11.7407) (7.3059, -11.7457) (7.3351, -11.7524) (7.3637, -11.7604) (7.392, -11.7697) (7.4198, -11.7809) (7.4473, -11.7935) (7.4746, -11.8077) (7.5017, -11.8238) (7.5285, -11.8417) (7.5554, -11.8613) (7.5818, -11.8829) (7.6083, -11.9058) (7.6254, -11.9223) (7.6341, -11.9307) knots 0 0 0 0 0.061617 0.122179 0.182216 0.241864 0.30096 0.359969 0.419033 0.478069 0.537993 0.59896 0.661321 0.725248 0.79122 0.858746 0.928318 1 1 1 1
  line L158 (7.6341, -11.9307) -> (7.5572, -12.0036)
  spline S161 degree 3 poles (7.5572, -12.0036) (7.5433, -11.9905) (7.5158, -11.9646) (7.4709, -11.931) (7.4241, -11.9023) (7.3756, -11.8789) (7.3266, -11.8602) (7.2778, -11.8469) (7.2296, -11.8384) (7.1976, -11.8374) (7.1818, -11.8369) knots 0 0 0 0 0.136144 0.269043 0.398517 0.5271 0.652283 0.77168 0.887495 1 1 1 1
  spline S162 degree 3 poles (7.1818, -11.8369) (7.1721, -11.837) (7.1527, -11.8373) (7.124, -11.8403) (7.0955, -11.8446) (7.0674, -11.8509) (7.0397, -11.8588) (7.0123, -11.8688) (6.9852, -11.8804) (6.9588, -11.8938) (6.9331, -11.9085) (6.9089, -11.9248) (6.886, -11.9421) (6.8647, -11.961) (6.845, -11.9812) (6.8265, -12.0024) (6.8097, -12.0251) (6.7945, -12.0489) (6.781, -12.0734) (6.7691, -12.0984) (6.759, -12.1237) (6.7511, -12.1495) (6.7445, -12.1755) (6.7399, -12.2018) (6.7373, -12.2286) (6.7369, -12.2466) (6.7367, -12.2556) knots 0 0 0 0 0.042841 0.085571 0.127719 0.170068 0.212787 0.255482 0.298877 0.342861 0.386528 0.429532 0.471886 0.513729 0.555082 0.596535 0.63812 0.679822 0.721331 0.761888 0.802199 0.841806 0.88106 0.920633 0.960101 1 1 1 1
  spline S163 degree 3 poles (6.7367, -12.2556) (6.7369, -12.2648) (6.7373, -12.2832) (6.7401, -12.3107) (6.7452, -12.3378) (6.752, -12.3645) (6.7606, -12.391) (6.7713, -12.4171) (6.7839, -12.4428) (6.7986, -12.4679) (6.8146, -12.4923) (6.8326, -12.5154) (6.8517, -12.5373) (6.8726, -12.5576) (6.8947, -12.5768) (6.9186, -12.5945) (6.9438, -12.6109) (6.9703, -12.6259) (6.998, -12.6393) (7.0264, -12.6512) (7.0555, -12.661) (7.0853, -12.6689) (7.1157, -12.6755) (7.1468, -12.6797) (7.1785, -12.6827) (7.1999, -12.683) (7.2106, -12.6831) knots 0 0 0 0 0.038994 0.077882 0.116652 0.155416 0.194618 0.234261 0.274547 0.315667 0.35702 0.398083 0.439098 0.479833 0.521274 0.562841 0.605292 0.648409 0.691727 0.735149 0.778369 0.821661 0.865524 0.909731 0.954523 1 1 1 1
  spline S164 degree 3 poles (7.2106, -12.6831) (7.2236, -12.6828) (7.249, -12.6823) (7.2865, -12.6781) (7.3224, -12.6717) (7.3568, -12.6622) (7.3896, -12.6501) (7.421, -12.6355) (7.4507, -12.6179) (7.4789, -12.598) (7.5048, -12.5759) (7.5282, -12.552) (7.5487, -12.5265) (7.5665, -12.4994) (7.5813, -12.4707) (7.5934, -12.4404) (7.6027, -12.4085) (7.6065, -12.3865) (7.6085, -12.3754) knots 0 0 0 0 0.07063 0.138694 0.204918 0.269441 0.332636 0.395302 0.457764 0.520657 0.582852 0.643315 0.70258 0.760908 0.81949 0.878269 0.938491 1 1 1 1
  line L159 (7.6085, -12.3754) -> (7.2751, -12.3754)
  line L160 (7.2751, -12.3754) -> (7.2751, -12.2728)
  line L161 (7.2751, -12.2728) -> (7.6982, -12.2728)
  spline S165 degree 3 poles (7.6982, -12.2728) (7.6977, -12.2919) (7.6968, -12.3294) (7.6901, -12.3839) (7.6793, -12.4354) (7.6645, -12.484) (7.6454, -12.5295) (7.6222, -12.572) (7.5944, -12.6113) (7.5631, -12.6476) (7.528, -12.68) (7.49, -12.7084) (7.4491, -12.7324) (7.4052, -12.7519) (7.3586, -12.7671) (7.3092, -12.7779) (7.2569, -12.7844) (7.2211, -12.7852) (7.2028, -12.7856) knots 0 0 0 0 0.071272 0.139493 0.204635 0.267406 0.328446 0.388397 0.447734 0.507392 0.566768 0.625478 0.684067 0.743248 0.804033 0.866499 0.931723 1 1 1 1
  spline S166 degree 3 poles (7.2028, -12.7856) (7.1915, -12.7855) (7.1693, -12.7852) (7.1364, -12.7829) (7.1044, -12.7794) (7.0733, -12.7741) (7.0431, -12.7676) (7.0137, -12.7593) (6.9853, -12.7497) (6.9576, -12.7387) (6.9309, -12.726) (6.9052, -12.7119) (6.8803, -12.6965) (6.8563, -12.6795) (6.8331, -12.661) (6.8109, -12.641) (6.7896, -12.6195) (6.7763, -12.6042) (6.7695, -12.5965) knots 0 0 0 0 0.069237 0.136557 0.202094 0.266464 0.329769 0.391879 0.453271 0.514115 0.57439 0.634142 0.693923 0.754152 0.81447 0.875661 0.937348 1 1 1 1
  spline S167 degree 3 poles (6.7695, -12.5965) (6.7598, -12.5843) (6.7404, -12.5602) (6.7154, -12.5214) (6.6942, -12.4813) (6.6769, -12.4397) (6.6635, -12.3967) (6.6538, -12.3522) (6.6482, -12.3064) (6.6473, -12.2753) (6.6469, -12.2596) knots 0 0 0 0 0.127896 0.253668 0.376738 0.499344 0.621999 0.745699 0.871345 1 1 1 1
  line L162 (7.9931, -11.9747) -> (7.9931, -12.76)
  line L163 (7.9931, -12.76) -> (7.9033, -12.76)
  line L164 (7.9033, -12.76) -> (7.9033, -11.76)
  line L165 (7.9033, -11.76) -> (7.9222, -11.76)
  line L166 (7.9222, -11.76) -> (8.5828, -12.5471)
  line L167 (8.5828, -12.5471) -> (8.5828, -11.76)
  line L168 (8.5828, -11.76) -> (8.6726, -11.76)
  line L169 (8.6726, -11.76) -> (8.6726, -12.76)
  line L170 (8.6726, -12.76) -> (8.6521, -12.76)
  line L171 (8.6521, -12.76) -> (7.9931, -11.9747)
  line L172 (3.179, -12.76) -> (3.5055, -12.25)
  line L173 (3.5055, -12.25) -> (3.1918, -11.76)
  line L174 (3.1918, -11.76) -> (3.2954, -11.76)
  line L175 (3.2954, -11.76) -> (3.5572, -12.1691)
  line L176 (3.5572, -12.1691) -> (3.819, -11.76)
  line L177 (3.819, -11.76) -> (3.9226, -11.76)
  line L178 (3.9226, -11.76) -> (3.6091, -12.25)
  line L179 (3.6091, -12.25) -> (3.9354, -12.76)
  line L180 (3.9354, -12.76) -> (3.8318, -12.76)
  line L181 (3.8318, -12.76) -> (3.5572, -12.3309)
  line L182 (3.5572, -12.3309) -> (3.2825, -12.76)
  line L183 (3.2825, -12.76) -> (3.179, -12.76)
  line L184 (2.8008, -12.76) -> (2.8008, -11.8626)
  line L185 (2.8008, -11.8626) -> (2.5828, -11.8626)
  line L186 (2.5828, -11.8626) -> (2.5828, -11.76)
  line L187 (2.5828, -11.76) -> (3.1085, -11.76)
  line L188 (3.1085, -11.76) -> (3.1085, -11.8626)
  line L189 (3.1085, -11.8626) -> (2.8905, -11.8626)
  line L190 (2.8905, -11.8626) -> (2.8905, -12.76)
  line L191 (2.8905, -12.76) -> (2.8008, -12.76)
  spline S168 degree 3 poles (9.7495, -12.2726) (9.7493, -12.285) (9.749, -12.3093) (9.7458, -12.3452) (9.7412, -12.3801) (9.734, -12.4137) (9.7253, -12.4463) (9.7142, -12.4777) (9.7014, -12.5081) (9.6866, -12.5371) (9.6702, -12.5645) (9.6527, -12.5904) (9.634, -12.6143) (9.614, -12.6364) (9.5928, -12.6566) (9.5704, -12.675) (9.5468, -12.6913) (9.5219, -12.7062) (9.4951, -12.7192) (9.466, -12.7302) (9.4342, -12.7393) (9.4001, -12.7469) (9.3633, -12.7529) (9.3241, -12.7569) (9.2823, -12.7596) (9.2536, -12.7599) (9.2389, -12.76) knots 0 0 0 0 0.046081 0.090807 0.134295 0.177024 0.218823 0.260244 0.30108 0.341614 0.381583 0.42012 0.458075 0.494738 0.531195 0.566934 0.602713 0.638327 0.674853 0.713467 0.754442 0.797815 0.843989 0.893072 0.944963 1 1 1 1
  line L192 (9.2389, -12.76) -> (8.929, -12.76)
  line L193 (8.929, -12.76) -> (8.929, -11.76)
  line L194 (8.929, -11.76) -> (9.1309, -11.76)
  spline S169 degree 3 poles (9.1309, -11.76) (9.1485, -11.7601) (9.1824, -11.7604) (9.2314, -11.7619) (9.2768, -11.7647) (9.3183, -11.7687) (9.3562, -11.7736) (9.3902, -11.7797) (9.4207, -11.7869) (9.4394, -11.7931) (9.4482, -11.7961) knots 0 0 0 0 0.164289 0.317406 0.458844 0.589367 0.707831 0.81577 0.91288 1 1 1 1
  spline S170 degree 3 poles (9.4482, -11.7961) (9.4598, -11.8005) (9.4827, -11.8092) (9.5152, -11.8256) (9.5459, -11.8443) (9.5748, -11.8651) (9.6013, -11.8888) (9.6265, -11.9142) (9.6492, -11.9424) (9.67, -11.9727) (9.6888, -12.0048) (9.7052, -12.0386) (9.7187, -12.0739) (9.73, -12.1107) (9.7388, -12.1491) (9.7449, -12.189) (9.7489, -12.2303) (9.7493, -12.2584) (9.7495, -12.2726) knots 0 0 0 0 0.061545 0.121694 0.181155 0.239875 0.298702 0.357647 0.417605 0.478494 0.540407 0.602345 0.665004 0.728559 0.793651 0.860534 0.929236 1 1 1 1
  line L195 (7.4931, -7.18) -> (7.5956, -6.68)
  line L196 (7.5956, -6.68) -> (8.0059, -6.68)
  line L197 (8.0059, -6.68) -> (8.0059, -6.7826)
  line L198 (8.0059, -6.7826) -> (7.6658, -6.7826)
  line L199 (7.6658, -6.7826) -> (7.6119, -7.0456)
  spline S171 degree 3 poles (7.6119, -7.0456) (7.6225, -7.0427) (7.643, -7.037) (7.6732, -7.0307) (7.702, -7.0269) (7.7206, -7.0264) (7.7297, -7.0262) knots 0 0 0 0 0.275068 0.532901 0.773973 1 1 1 1
  spline S172 degree 3 poles (7.7297, -7.0262) (7.7408, -7.0264) (7.7628, -7.0269) (7.7949, -7.0314) (7.8256, -7.0386) (7.8547, -7.0487) (7.8824, -7.0615) (7.9083, -7.0775) (7.933, -7.0962) (7.9558, -7.1178) (7.9765, -7.1415) (7.9947, -7.1669) (8.0102, -7.1939) (8.0227, -7.2227) (8.0326, -7.253) (8.0392, -7.2851) (8.0436, -7.3186) (8.0441, -7.3416) (8.0444, -7.3533) knots 0 0 0 0 0.065808 0.129394 0.190894 0.251281 0.310815 0.370371 0.430768 0.492881 0.555104 0.616067 0.677256 0.73826 0.800762 0.864778 0.931045 1 1 1 1
  spline S173 degree 3 poles (8.0444, -7.3533) (8.0442, -7.3614) (8.0438, -7.3776) (8.0419, -7.4017) (8.0382, -7.4252) (8.0332, -7.4482) (8.0268, -7.4707) (8.019, -7.4927) (8.0094, -7.5141) (7.999, -7.535) (7.9872, -7.5551) (7.9741, -7.5738) (7.9603, -7.5916) (7.9454, -7.6081) (7.9294, -7.6233) (7.9123, -7.6373) (7.8944, -7.6503) (7.8754, -7.6618) (7.8556, -7.6723) (7.8348, -7.681) (7.8136, -7.6887) (7.7915, -7.6949) (7.7686, -7.6997) (7.7449, -7.703) (7.7205, -7.7054) (7.704, -7.7056) (7.6956, -7.7056) knots 0 0 0 0 0.044014 0.087434 0.130118 0.172554 0.214555 0.256298 0.298438 0.340849 0.382715 0.423924 0.464246 0.504074 0.543862 0.583567 0.623094 0.663229 0.703551 0.743938 0.784541 0.82575 0.867757 0.910745 0.954914 1 1 1 1
  spline S174 degree 3 poles (7.6956, -7.7056) (7.6856, -7.7054) (7.666, -7.7051) (7.6373, -7.701) (7.6097, -7.6952) (7.5834, -7.6864) (7.5581, -7.6755) (7.5343, -7.6616) (7.5112, -7.6459) (7.49, -7.6273) (7.4702, -7.6071) (7.4525, -7.5851) (7.4368, -7.5617) (7.4232, -7.5369) (7.4116, -7.5107) (7.4025, -7.4829) (7.3952, -7.4538) (7.3921, -7.4338) (7.3905, -7.4236) knots 0 0 0 0 0.065421 0.128708 0.190236 0.250724 0.310637 0.370766 0.431615 0.493523 0.555883 0.617342 0.678668 0.740711 0.802985 0.866803 0.932347 1 1 1 1
  line L200 (7.3905, -7.4236) -> (7.4803, -7.4236)
  spline S175 degree 3 poles (7.4803, -7.4236) (7.4825, -7.4331) (7.4867, -7.4515) (7.496, -7.4772) (7.5074, -7.5002) (7.521, -7.5206) (7.5371, -7.5384) (7.5556, -7.5543) (7.5762, -7.5687) (7.5992, -7.5806) (7.6234, -7.5908) (7.6488, -7.5976) (7.6746, -7.6024) (7.692, -7.6028) (7.7008, -7.6031) knots 0 0 0 0 0.094687 0.181994 0.264377 0.34218 0.418618 0.496509 0.577369 0.661511 0.746733 0.831258 0.915206 1 1 1 1
  spline S176 degree 3 poles (7.7008, -7.6031) (7.7094, -7.6028) (7.7262, -7.6024) (7.751, -7.5988) (7.775, -7.5934) (7.7978, -7.5852) (7.82, -7.5752) (7.8409, -7.5624) (7.8612, -7.5477) (7.8801, -7.5309) (7.8975, -7.5123) (7.9129, -7.4925) (7.9257, -7.4713) (7.9364, -7.4492) (7.9446, -7.4258) (7.9505, -7.4014) (7.9539, -7.3758) (7.9544, -7.3584) (7.9546, -7.3495) knots 0 0 0 0 0.064207 0.126425 0.18768 0.248216 0.308305 0.369661 0.431699 0.495947 0.559758 0.622295 0.683911 0.745092 0.80674 0.869087 0.93329 1 1 1 1
  spline S177 degree 3 poles (7.9546, -7.3495) (7.9544, -7.3414) (7.9541, -7.3257) (7.9511, -7.3028) (7.9458, -7.281) (7.9386, -7.2604) (7.9293, -7.2409) (7.9181, -7.2225) (7.9045, -7.2055) (7.8891, -7.1897) (7.8721, -7.1752) (7.8534, -7.1628) (7.8334, -7.1524) (7.8122, -7.1434) (7.7893, -7.137) (7.7653, -7.1321) (7.7398, -7.1293) (7.7224, -7.1289) (7.7134, -7.1287) knots 0 0 0 0 0.065351 0.127916 0.18836 0.247216 0.30563 0.36377 0.422661 0.482687 0.5433 0.604118 0.664965 0.727413 0.791468 0.858055 0.927037 1 1 1 1
  spline S178 degree 3 poles (7.7134, -7.1287) (7.7057, -7.1289) (7.6897, -7.1292) (7.6651, -7.1317) (7.6393, -7.1358) (7.6124, -7.1414) (7.5842, -7.1487) (7.5549, -7.1575) (7.5243, -7.168) (7.5037, -7.1759) (7.4931, -7.18) knots 0 0 0 0 0.102203 0.211023 0.3251 0.446502 0.573788 0.708901 0.850358 1 1 1 1
  spline S179 degree 3 poles (7.1854, -6.9596) (7.1852, -6.9528) (7.1848, -6.9394) (7.1817, -6.9197) (7.1769, -6.9006) (7.1701, -6.8823) (7.161, -6.8647) (7.15, -6.848) (7.1374, -6.8318) (7.1227, -6.8166) (7.1066, -6.8027) (7.0895, -6.7903) (7.0715, -6.78) (7.0526, -6.7716) (7.0328, -6.765) (7.0121, -6.7604) (6.9906, -6.7575) (6.9759, -6.7571) (6.9684, -6.7569) knots 0 0 0 0 0.061965 0.122122 0.180988 0.239933 0.299906 0.359989 0.421776 0.486576 0.551535 0.615018 0.677259 0.73973 0.80305 0.866495 0.931973 1 1 1 1
  spline S180 degree 3 poles (6.9684, -6.7569) (6.9606, -6.7571) (6.9453, -6.7575) (6.9227, -6.7603) (6.9012, -6.7652) (6.8807, -6.7718) (6.8611, -6.7802) (6.8426, -6.7907) (6.8251, -6.8032) (6.8087, -6.8174) (6.7936, -6.8332) (6.7804, -6.8508) (6.7688, -6.8699) (6.7586, -6.8904) (6.7504, -6.9126) (6.7441, -6.9363) (6.7392, -6.9614) (6.7375, -6.9788) (6.7367, -6.9877) knots 0 0 0 0 0.064439 0.126547 0.186887 0.245878 0.304041 0.362191 0.420976 0.48066 0.5406 0.600689 0.661936 0.724443 0.789038 0.856314 0.926352 1 1 1 1
  line L201 (6.7367, -6.9877) -> (6.6469, -6.9877)
  spline S181 degree 3 poles (6.6469, -6.9877) (6.6475, -6.9758) (6.6487, -6.9524) (6.654, -6.9183) (6.6617, -6.8857) (6.6726, -6.8549) (6.6861, -6.8256) (6.7023, -6.7979) (6.7215, -6.7719) (6.7433, -6.7478) (6.767, -6.7258) (6.7925, -6.7067) (6.8193, -6.6906) (6.8473, -6.6772) (6.8769, -6.6671) (6.9077, -6.6596) (6.9399, -6.6551) (6.9619, -6.6546) (6.973, -6.6544) knots 0 0 0 0 0.068791 0.135103 0.198979 0.261904 0.323495 0.385195 0.446969 0.509765 0.572251 0.633405 0.693251 0.752583 0.812579 0.873275 0.93555 1 1 1 1
  spline S182 degree 3 poles (6.973, -6.6544) (6.984, -6.6546) (7.0056, -6.6551) (7.037, -6.6595) (7.0669, -6.6662) (7.0953, -6.6758) (7.1219, -6.6886) (7.1469, -6.7039) (7.1705, -6.7217) (7.1919, -6.7426) (7.2114, -6.765) (7.2283, -6.7888) (7.2428, -6.8135) (7.2548, -6.8391) (7.2637, -6.8659) (7.2704, -6.8935) (7.2742, -6.9223) (7.2748, -6.9417) (7.2751, -6.9516) knots 0 0 0 0 0.069475 0.136517 0.200789 0.26383 0.325735 0.387291 0.449509 0.512968 0.576275 0.63758 0.697903 0.757172 0.816599 0.876653 0.93729 1 1 1 1
  spline S183 degree 3 poles (7.2751, -6.9516) (7.2746, -6.9656) (7.2737, -6.9932) (7.2655, -7.0337) (7.2527, -7.0731) (7.2372, -7.1047) (7.2217, -7.1302) (7.2077, -7.1512) (7.1912, -7.1738) (7.1722, -7.1979) (7.1509, -7.2238) (7.1272, -7.2514) (7.1009, -7.2803) (7.0824, -7.3001) (7.0728, -7.3104) knots 0 0 0 0 0.098702 0.195672 0.292422 0.391343 0.444462 0.504229 0.570352 0.642546 0.722288 0.807921 0.90047 1 1 1 1
  line L202 (7.0728, -7.3104) -> (6.8226, -7.5774)
  line L203 (6.8226, -7.5774) -> (7.2879, -7.5774)
  line L204 (7.2879, -7.5774) -> (7.2879, -7.68)
  line L205 (7.2879, -7.68) -> (6.6085, -7.68)
  line L206 (6.6085, -7.68) -> (6.9963, -7.2661)
  spline S184 degree 3 poles (6.9963, -7.2661) (7.0057, -7.2563) (7.0239, -7.2373) (7.0495, -7.2097) (7.0726, -7.1841) (7.0931, -7.1605) (7.1108, -7.1386) (7.1265, -7.1191) (7.139, -7.1012) (7.1527, -7.0804) (7.1659, -7.055) (7.1772, -7.024) (7.1841, -6.9921) (7.185, -6.9705) (7.1854, -6.9596) knots 0 0 0 0 0.110803 0.212829 0.306101 0.390647 0.466924 0.534481 0.593587 0.644557 0.7362 0.825024 0.911986 1 1 1 1
  spline S185 degree 3 poles (3.9546, -6.9596) (3.9544, -6.9528) (3.9541, -6.9394) (3.9509, -6.9197) (3.9461, -6.9006) (3.9393, -6.8823) (3.9303, -6.8647) (3.9193, -6.848) (3.9066, -6.8318) (3.8919, -6.8166) (3.8758, -6.8027) (3.8588, -6.7903) (3.8408, -6.78) (3.8218, -6.7716) (3.8021, -6.765) (3.7814, -6.7604) (3.7599, -6.7575) (3.7452, -6.7571) (3.7377, -6.7569) knots 0 0 0 0 0.061965 0.122122 0.180988 0.239933 0.299906 0.359989 0.421776 0.486576 0.551535 0.615018 0.677259 0.73973 0.80305 0.866495 0.931973 1 1 1 1
  spline S186 degree 3 poles (3.7377, -6.7569) (3.7298, -6.7571) (3.7145, -6.7575) (3.6919, -6.7603) (3.6704, -6.7652) (3.6499, -6.7718) (3.6303, -6.7802) (3.6118, -6.7907) (3.5943, -6.8032) (3.578, -6.8174) (3.5629, -6.8332) (3.5496, -6.8508) (3.538, -6.8699) (3.5279, -6.8904) (3.5197, -6.9126) (3.5134, -6.9363) (3.5084, -6.9614) (3.5067, -6.9788) (3.5059, -6.9877) knots 0 0 0 0 0.064439 0.126547 0.186887 0.245878 0.304041 0.362191 0.420976 0.48066 0.5406 0.600689 0.661936 0.724443 0.789038 0.856314 0.926352 1 1 1 1
  line L207 (3.5059, -6.9877) -> (3.4162, -6.9877)